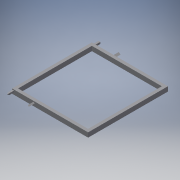
# Autodesk Inventor part: Zijplaat 1.1
Saved by Autodesk Inventor 2018.3 (Build 223284000, 284)
## iProperties
Created: 2020-11-16
Part Number: Zijplaat 1.1
Material: Generic
Document SubType Name: Modeling
Designer: daanv
Density: 1 g/cm^3
Appearance: Default
Author: daanv
Autodesk Inventor part; units mm, degrees
ref_plane "YZ Plane" through (0, 0, 0) normal (1, 0, 0) x (0, 1, 0)
ref_plane "XZ Plane" through (0, 0, 0) normal (0, 1, 0) x (-1, 0, 0)
ref_plane "XY Plane" through (0, 0, 0) normal (0, 0, 1) x (1, 0, 0)
sketch "Sketch1" plane through (0, 0, 0) normal (0, 0, 1) x (1, 0, 0)
  line L0 (0, 0) -> (50, 0)
  line L1 (50, 0) -> (50, 52.5)
  line L2 (50, 52.5) -> (0, 52.5)
  line L3 (0, 52.5) -> (0, 0)
  dimension "d0" = 50
  dimension "d1" = 52.5
  constraints: 8 end point, 2 parallel, 1 horizontal, 1 perpendicular
  measures "d0" distance of L2.end L1.end
  measures "d1" distance of L1.end L0.end
extrude "Extrusion1" add sketch "Sketch1" along normal blind 3
sketch "Sketch2" plane through (0, 0, 3) normal (0, 0, 1) x (1, 0, 0)
  line L0 (2, 50.5) -> (48, 50.5)
  line L1 (48, 50.5) -> (48, 2)
  line L2 (48, 2) -> (2, 2)
  line L3 (2, 2) -> (2, 50.5)
  dimension "d4" = 46
  dimension "d5" = 48.5
  constraints: 8 end point, 2 parallel, 1 horizontal, 1 perpendicular
  measures "d4" distance of L1.end L2.end
  measures "d5" distance of L0.end L1.end
extrude "Extrusion2" cut sketch "Sketch2" against normal blind 10
sketch "Sketch5" plane through (0, 0, 0) normal (0, -1, 0) x (1, 0, 0)
  line L0 (12.85, 2.5) -> (12.85, 1.5) projected
  line L1 (2.85, 1.5) -> (2.85, 2.5) projected
  line L2 (0, 0) -> (50, 0) projected
  line L3 (14.1, 2.5) -> (14.966, 2)
  line L4 (14.966, 2) -> (14.1, 1.5)
  line L5 (14.1, 1.5) -> (14.1, 2.5)
  line L6 (2, 3) -> (48, 3) projected
  line L7 (1.35, 2.5) -> (0.35, 2.5)
  line L8 (0.35, 2.5) -> (0.35, 1.5)
  line L9 (0.35, 1.5) -> (1.35, 1.5)
  line L10 (1.35, 1.5) -> (1.35, 2.5)
  dimension "d24" = 1
  dimension "d25" = 1
  dimension "d26" = 1.5
  dimension "d27" = 1.25
  dimension "d28" = 1
  dimension "d29" = 1
  dimension "d30" = 1
  dimension "d31" = 1
  dimension "d32" = 1
  dimension "d33" = 0.5
  dimension "d34" = 1.5
  constraints: 14 end point, 4 perpendicular, 1 horizontal
  measures "d24" distance of L3.start L3.end
  measures "d25" distance of L7.start L7.end
  measures "d26" distance between parallel lines of L10 L1
  measures "d27" distance between parallel lines of L0 L5
  measures "d28" distance of L8.end L9.end
  measures "d29" distance of L7.end L8.end
  measures "d30" distance of L9.end L7.start
  measures "d31" distance of L3.end L4.end
  measures "d32" distance of L4.end L3.start
  measures "d33" distance from line of L6 L3.start
  measures "d34" distance between parallel lines of L2 L9
extrude "Extrusion5" add sketch "Sketch5" along normal blind 4
chamfer "Chamfer3" distance 0.288 angle 45 3 edges at (14.533, -4, 1.75) (14.1, -4, 2) (14.533, -4, 2.25)
chamfer "Chamfer4" distance 0.288 angle 45 3 edges at (14.533, -3.712, 1.75) (14.1, -3.712, 2) (14.533, -3.712, 2.25)
chamfer "Chamfer5" distance 0.499 angle 45 4 edges at (0.85, -4, 1.5) (1.35, -4, 2) (0.85, -4, 2.5) (0.35, -4, 2)
chamfer "Chamfer6" distance 0.499 angle 45 4 edges at (0.85, -3.501, 1.5) (1.35, -3.501, 2) (0.85, -3.501, 2.5) (0.35, -3.501, 2)
sketch "Sketch8" plane through (0, 52.5, 0) normal (0, 1, 0) x (1, 0, 0)
  line L0 (50, 0) -> (0, 0) projected
  line L1 (50, 0) -> (50, -3) projected
  line L2 (13.7626, -1) -> (14.6286, -1.5)
  line L3 (13.7626, -1) -> (14.7626, -1) construction
  line L4 (14.6286, -1.5) -> (13.7626, -2)
  line L5 (12.66, -2.77) -> (12.66, -0.23) projected
  line L6 (13.7626, -2) -> (13.7626, -1)
  line L7 (13.5765, -2.1075) -> (13.5765, -0.8925)
  line L8 (13.5765, -0.8925) -> (13.5765, -0.7425)
  line L9 (13.5765, -0.7425) -> (14.8884, -1.5)
  line L10 (13.5765, -2.1075) -> (13.5765, -2.2575)
  line L11 (13.5765, -2.2575) -> (14.8884, -1.5)
  dimension "d60" = 1
  dimension "d61" = 30
  dimension "d62" = 1
  dimension "d63" = 60
  dimension "d64" = 1
  dimension "d65" = 35.3714
  dimension "d66" = 0.15
  dimension "d67" = 60
  dimension "d68" = 0.15
  constraints: 18 end point, 2 vertical, 1 equal length, 1 horizontal, 1 point on line
  measures "d60" distance of L2.start L2.end
  measures "d61" angle of L2 L3
  measures "d62" distance of L2.end L4.end
  measures "d63" angle of L2 L4
  measures "d64" distance from line of L0 L2.start
  measures "d65" distance from line of L1 L2.end
  measures "d66" distance of L7.end L8.end
  measures "d67" angle of L8 L9
  measures "d68" distance of L7.start L10.end
extrude "Extrusion8" add sketch "Sketch8" along normal blind 4
chamfer "Chamfer7" distance 0.12 angle 45 3 edges at (14.1956, 56.5, 1.75) (13.7626, 56.5, 1.5) (14.1956, 56.5, 1.25)
sketch "Sketch9" plane through (0, 52.5, 0) normal (0, 1, 0) x (1, 0, 0)
  line L0 (50, 0) -> (0, 0) projected
  line L1 (0, 0) -> (0, -3) projected
  line L2 (50, -3) -> (0, -3) projected
  line L3 (2, -2.77) -> (2, -0.23) projected
  line L4 (1.5, -2) -> (0.5, -2)
  line L5 (0.5, -2) -> (0.5, -1)
  line L6 (0.5, -1) -> (1.5, -1)
  line L7 (1.5, -1) -> (1.5, -2)
  line L8 (1.6, -2.1) -> (0.4, -2.1)
  line L9 (0.4, -2.1) -> (0.4, -0.9)
  line L10 (0.4, -0.9) -> (1.6, -0.9)
  line L11 (1.6, -0.9) -> (1.6, -2.1)
  dimension "d74" = 1
  dimension "d75" = 1
  dimension "d76" = 0.5
  dimension "d77" = 1
  dimension "d78" = 1
  dimension "d79" = 0.5
  dimension "d81" = 1.2
  dimension "d82" = 1.2
  constraints: 16 end point, 4 parallel, 2 horizontal, 2 perpendicular
  measures "d74" distance of L5.end L6.end
  measures "d75" distance of L4.end L5.end
  measures "d76" distance between parallel lines of L3 L7
  measures "d77" distance between parallel lines of L2 L4
  measures "d78" distance between parallel lines of L0 L6
  measures "d79" distance between parallel lines of L1 L5
  measures "d81" distance of L9.end L10.end
  measures "d82" distance of L8.end L9.end
extrude "Extrusion9" add sketch "Sketch9" along normal blind 4
chamfer "Chamfer8" distance 0.1 angle 45 4 edges at (1.5, 56.5, 1.5) (1, 56.5, 2) (0.5, 56.5, 1.5) (1, 56.5, 1)
chamfer "Chamfer9" distance 0.1 angle 45 4 edges at (0.5, 56.4005, 1.5) (1, 56.4005, 2) (1.5, 56.4005, 1.5) (1, 56.4005, 1)
chamfer "Chamfer10" distance 0.1 angle 45 3 edges at (14.1956, 56.38, 1.75) (13.7626, 56.38, 1.5) (14.1956, 56.38, 1.25)
body "Solid1"
